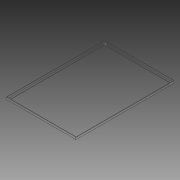
# Autodesk Inventor part: Chassis
Saved by Autodesk Inventor 2015 (Build 190159000, 159)
## iProperties
Created: 2016-02-06
Part Number: Chassis
Material: Generic
Document SubType Name: Modeling
Designer: sethbattis
Density: 1 g/cm^3
Appearance: Default
Author: sethbattis
Autodesk Inventor part; units mm, degrees
ref_plane "YZ Plane" through (0, 0, 0) normal (1, 0, 0) x (0, 1, 0)
ref_plane "XZ Plane" through (0, 0, 0) normal (0, 1, 0) x (-1, 0, 0)
ref_plane "XY Plane" through (0, 0, 0) normal (0, 0, 1) x (1, 0, 0)
sketch "Sketch1" plane through (0, 0, 0) normal (0, 0, 1) x (1, 0, 0)
  line L0 (292.1, 0) -> (292.1, 3.175)
  line L1 (292.1, 3.175) -> (307.975, 3.175)
  line L2 (307.975, 3.175) -> (307.975, 19.05)
  line L3 (307.975, 19.05) -> (311.15, 19.05)
  line L4 (311.15, 19.05) -> (311.15, 0)
  line L5 (311.15, 0) -> (292.1, 0)
  line L6 (-435.61, 0) -> (435.61, 0) construction
  line L7 (0, -3.81) -> (0, 22.86) construction
  line L8 (-292.1, 0) -> (-292.1, 3.175)
  line L9 (-292.1, 3.175) -> (-307.975, 3.175)
  line L10 (-307.975, 3.175) -> (-307.975, 19.05)
  line L11 (-307.975, 19.05) -> (-311.15, 19.05)
  line L12 (-311.15, 19.05) -> (-311.15, 0)
  line L13 (-311.15, 0) -> (-292.1, 0)
  point P0 (0, 0)
  dimension "d4" = 19.05
  dimension "d5" = 3.175
  dimension "d6" = 622.3
  constraints: 24 end point, 9 perpendicular, 6 equal length, 2 collinear, 2 point on line, 2 vertical, 1 other
  measures "d4" distance of L4.end L0.start
  measures "d5" distance of L0.start L0.end
  measures "d6" distance between parallel lines of L4 L12
extrude "Extrusion2" add sketch "Sketch1" along normal blind 876.3
sketch "Sketch2" plane through (-307.975, 19.05, 876.3) normal (1, 0, 0) x (0, 0, -1)
  line L0 (876.3, -15.875) -> (0, -15.875) projected
  line L1 (19.05, -15.875) -> (19.05, -12.7)
  line L2 (19.05, -12.7) -> (3.175, -12.7)
  line L3 (3.175, -12.7) -> (3.175, 3.175)
  line L4 (3.175, 3.175) -> (0, 3.175)
  line L5 (0, 3.175) -> (0, -15.875)
  line L6 (0, -15.875) -> (0, 0) projected
  line L7 (0, -15.875) -> (19.05, -15.875)
  line L8 (0, -15.875) -> (19.05, -15.875)
  line L9 (857.25, -15.875) -> (857.25, -12.7)
  line L10 (857.25, -12.7) -> (873.125, -12.7)
  line L11 (873.125, -12.7) -> (873.125, 3.175)
  line L12 (873.125, 3.175) -> (876.3, 3.175)
  line L13 (876.3, 3.175) -> (876.3, -15.875)
  line L14 (857.25, -15.875) -> (876.3, -15.875)
  line L15 (0, -19.05) -> (0, 0) projected
  point P0 (876.3, -19.05)
  dimension "d9" = 3.175
  dimension "d10" = 19.05
  constraints: 26 end point, 8 perpendicular, 6 equal length, 3 collinear, 2 point on line, 2 vertical
  measures "d9" distance of L1.start L1.end
  measures "d10" distance of L4.end L0.end
extrude "Extrusion3" add sketch "Sketch2" along normal up to surface (615.95 mm away)
body "Solid2"
